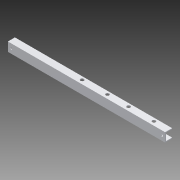
# Autodesk Inventor part: 26in C-Channel Right
Saved by Autodesk Inventor 2013 (Build 170138000, 138)
## iProperties
Created: 2013-01-08
Part Number: 26in C-Channel Right
Material: Aluminum 6061
Document SubType Name: Modeling
Designer: Naphat
Density: 2.71 g/cm^3
Mass: 341.078 g
Surface Area: 882.87 cm^2
Volume: 125.859 cm^3
Author: Naphat
Autodesk Inventor part; units mm, degrees
ref_plane "YZ Plane" through (0, 0, 0) normal (1, 0, 0) x (0, 1, 0)
ref_plane "XZ Plane" through (0, 0, 0) normal (0, 1, 0) x (-1, 0, 0)
ref_plane "XY Plane" through (0, 0, 0) normal (0, 0, 1) x (1, 0, 0)
sketch "Sketch1" plane through (0, 0, 0) normal (0, 0, 1) x (1, 0, 0)
  line L0 (-16, 12.5) -> (-13, 12.5)
  line L1 (-13, 12.5) -> (-13, -9.5)
  line L2 (-13, -9.5) -> (13, -9.5)
  line L3 (13, -9.5) -> (13, 12.5)
  line L4 (13, 12.5) -> (16, 12.5)
  line L5 (16, 12.5) -> (16, -12.5)
  line L6 (16, -12.5) -> (-16, -12.5)
  line L7 (-16, -12.5) -> (-16, 12.5)
  point P0 (0, 0)
  dimension "d0" = 3
  dimension "d2" = 3
  dimension "d3" = 25
  dimension "d4" = 32
  dimension "d5" = 16
  dimension "d7" = 12.5
  dimension "d8" = 3
  dimension "d74" = 25
  constraints: 16 end point, 5 parallel, 1 collinear, 1 horizontal, 1 perpendicular
  measures "d0" distance of L0.start L0.end
  measures "d2" distance of L3.end L4.end
  measures "d3" distance of L6.end L0.start
  measures "d4" distance of L5.end L6.end
  measures "d5" distance from line of point (0, 0) L7
  measures "d7" distance from line of L6 point (0, 0)
  measures "d8" distance between parallel lines of L6 L2
  measures "d74" distance between parallel lines of L6 L4
extrude "Extrusion1" add sketch "Sketch1" against normal blind 558.8
sketch "Sketch8" plane through (-16, -12.5, 0) normal (0, -1, 0) x (1, 0, 0)
  line L0 (32, -558.8) -> (0, -558.8) projected
  line L1 (32, 0) -> (32, -558.8) projected
  circle A0 centre (16, -547.8) radius 3.175
  line L2 (32, 0) -> (0, 0) projected
  circle A1 centre (16, -11) radius 3.175
  point P0 (16, 0)
  dimension "d114" = 6.35
  dimension "d116" = 16
  dimension "d117" = 11
  dimension "d125" = 6.35
  dimension "d126" = 11
  constraints: 2 centre point
  measures "d114" diameter of A0
  measures "d116" distance from line of A0.centre L1
  measures "d117" distance from line of A0.centre L0
  measures "d125" diameter of A1
  measures "d126" distance from line of A1.centre L2
hole "Hole5" at (0, -12.5, -547.8) at (0, -12.5, -11) direction (0, 1, 0) diameter 6.35 end through all
sketch "Sketch9" plane through (-13, -9.5, 0) normal (1, 0, 0) x (0, 0, -1)
  line L0 (0, 0) -> (558.8, 0) projected
  line L1 (0, 22) -> (558.8, 22) projected
  line L2 (-3, -6) -> (-3, 26) construction
  line L3 (98.6, 0) -> (98.6, 22) construction
  circle A0 centre (143.6, 11) radius 6
  circle A1 centre (53.6, 11) radius 6
  line L4 (263.7, 0) -> (263.7, 22) construction
  circle A2 centre (218.7, 11) radius 6
  circle A3 centre (308.7, 11) radius 6
  point P0 (0, 9.5)
  dimension "d127" = 101.6
  dimension "d128" = 12
  dimension "d129" = 12
  dimension "d130" = 11
  dimension "d132" = 90
  dimension "d133" = 45
  dimension "d134" = 165.1
  dimension "d135" = 12
  dimension "d136" = 12
  dimension "d137" = 90
  dimension "d138" = 45
  constraints: 4 centre point, 4 end point, 4 point on line, 3 horizontal alignment, 1 parallel, 1 perpendicular
  measures "d127" distance between parallel lines of L2 L3
  measures "d128" diameter of A0
  measures "d129" diameter of A1
  measures "d130" distance from line of L1 A1.centre
  measures "d132" distance of A0.centre A1.centre
  measures "d133" distance from line of A0.centre L3
  measures "d134" distance between parallel lines of L3 L4
  measures "d135" diameter of A2
  measures "d136" diameter of A3
  measures "d137" distance of A3.centre A2.centre
  measures "d138" distance from line of L4 A3.centre
hole "Hole6" at (-13, 1.5, -308.7) at (-13, 1.5, -218.7) at (-13, 1.5, -143.6) at (-13, 1.5, -53.6) direction (-1, 0, 0) diameter 12 depth 3 tip angle 118
equation "\"d2\" = d0"
equation "\"d5\" = 0.5 * d4"
equation "\"d7\" = 0.5 * d3"
equation "\"d8\" = d0"
equation "\"d74\" = d3"
equation "\"d126\" = d117"
equation "\"d133\" = 0.5 * d132"
equation "\"d137\" = d132"
equation "\"d138\" = d133"
body "Solid1"
